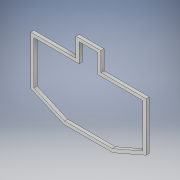
# Autodesk Inventor part: Buste2
Saved by Autodesk Inventor 2018 (Build 220112000, 112)
## iProperties
Created: 2018-02-13
Part Number: Buste2
Material: Generic
Document SubType Name: Modeling
Designer: Lilia
Density: 1 g/cm^3
Appearance: Default
Author: Lilia
Autodesk Inventor part; units mm, degrees
ref_plane "YZ Plane" through (0, 0, 0) normal (1, 0, 0) x (0, 1, 0)
ref_plane "XZ Plane" through (0, 0, 0) normal (0, 1, 0) x (-1, 0, 0)
ref_plane "XY Plane" through (0, 0, 0) normal (0, 0, 1) x (1, 0, 0)
sketch "Sketch1" plane through (0, 0, 0) normal (0, 0, 1) x (1, 0, 0)
  line L0 (-107.9, 41.925) -> (107.9, -41.925) construction
  line L1 (107.9, 41.925) -> (-107.9, -41.925) construction
  line L2 (-114.4, -47.125) -> (-114.4, 47.125)
  line L3 (114.4, 47.125) -> (114.4, -47.125)
  line L4 (114.4, -47.125) -> (-114.4, 47.125) construction
  line L5 (-114.4, -47.125) -> (114.4, 47.125) construction
  line L6 (-22.1, 47.125) -> (-22.1, 86.125)
  line L7 (-22.1, 86.125) -> (22.1, 86.125)
  line L8 (22.1, 86.125) -> (22.1, 47.125)
  line L9 (22.1, 47.125) -> (114.4, 47.125)
  line L10 (-22.1, 47.125) -> (-114.4, 47.125)
  line L11 (114.4, -47.125) -> (49.4, -75.4283)
  line L12 (-114.4, -47.125) -> (-49.4, -75.4283)
  line L13 (49.4, -75.4283) -> (-49.4, -75.4283)
  point P0 (0, 0)
  point P1 (0, 0)
  point P2 (0, 80.925)
  point P3 (0, 0)
  point P4 (0, 86.125)
  point P5 (0, 0)
  dimension "Comp" = 215.8
  dimension "Lar" = 83.85
  dimension "d10" = 215.8
  dimension "LarMaior" = 94.25
  dimension "CompMaior" = 228.8
  dimension "d20" = 39
  dimension "d21" = 44.2
  dimension "d25" = 65
  dimension "d27" = 65
  dimension "d28" = 98.8
  constraints: 28 end point, 8 midpoint, 3 equal length, 2 vertical alignment, 1 point on line
  measures "Comp" distance of L0.start L1.start
  measures "Lar" distance of L1.end L0.start
  measures "d10" distance of L0.end L1.end
  measures "LarMaior" distance of L3.start L3.end
  measures "CompMaior" distance of L2.end L3.start
  measures "d20" distance of L7.end L8.end
  measures "d21" distance of L6.end L7.end
  measures "d25" horizontal distance of L3.end L11.end
  measures "d27" horizontal distance of L2.start L12.end
  measures "d28" distance of L11.end L12.end
extrude "Extrusion1" add sketch "Sketch1" along normal blind 6.5
shell "Shell1" thickness 6.5 both sides yes removed faces 2 at (-7.3667, -34.5772, 6.5) at (-7.3667, -34.5772, 0)
body "Solid1"
